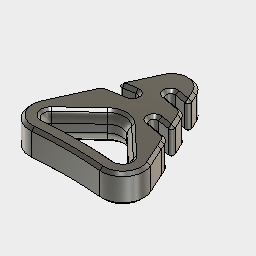
GuylineQuickAdjuster (Autodesk Fusion 360 design; units mm, degrees)
Autodesk Fusion 360 part; units mm, degrees
sketch "Sketch1" plane through (0, 0, 0) normal (0, 0, 1) x (1, 0, 0)
  line L0 (6.8861, 1.5182) -> (1.7133, 6.3871)
  line L1 (8.5, 0) -> (18.6301, 0) construction
  line L2 (-6.8869, 1.5182) -> (-1.7136, 6.3872)
  arc A0 (6.3068, 0.2249) -> (-6.3077, 0.2249) centre (-0.0001, -72) ccw
  arc A1 (-6.8869, 1.5182) -> (-6.3077, 0.2249) centre (-6.3729, 0.972) ccw
  arc A2 (6.3068, 0.2249) -> (6.8861, 1.5182) centre (6.372, 0.9721) ccw
  arc A3 (1.7133, 6.3871) -> (-1.7136, 6.3872) centre (-0.0002, 4.5667) ccw
  arc A4 (-9.7878, 2.5199) -> (-6.0467, -2.7631) centre (-6.3729, 0.972) ccw
  arc A5 (6.0459, -2.763) -> (-6.0467, -2.7631) centre (-0.0001, -72) ccw
  arc A6 (6.0459, -2.763) -> (9.7871, 2.5196) centre (6.372, 0.9721) ccw
  line L3 (-0.0001, 7.0667) -> (-0.0001, 7.5)
  line L4 (-0.0001, 7.0667) -> (-0.0027, 10.0001) construction
  line L5 (-0.0027, 10.0001) -> (-0.0001, 12.0001) construction
  line L6 (-0.0001, 12.0001) -> (0.0118, 15.0001) construction
  line L7 (0.0118, 15.0001) -> (6.9911, 13.7685) construction
  line L8 (-0.0027, 10.0001) -> (11.5438, 7.9642) construction
  line L9 (-0.0027, 10.0001) -> (11.5483, 10.0001) construction
  line L10 (-0.0001, 12.0001) -> (-12.6146, 9.7758) construction
  line L11 (-0.0001, 12.0001) -> (12.8092, 12.0001) construction
  line L12 (-4.6584, 11.9394) -> (-2.6377, 12.2955)
  line L13 (-2.3804, 10.8188) -> (-5.3051, 10.3031)
  line L14 (-6.7795, 9.159) -> (-9.7878, 2.5199)
  line L15 (8.2551, 5.8972) -> (9.7871, 2.5196)
  line L16 (-0.1302, 14.2615) -> (0, 14.2386)
  line L17 (0.9018, 14.0794) -> (3.819, 13.5647)
  arc A7 (-2.3804, 10.8188) -> (-2.6377, 12.2955) centre (-2.5076, 11.5574) ccw
  arc A8 (-5.2006, 12.6383) -> (-4.6584, 11.9394) centre (-4.7452, 12.4318) ccw
  arc A9 (-5.3051, 10.3031) -> (-6.7795, 9.159) centre (-4.9578, 8.3335) ccw
  arc A10 (5.2925, 12.4219) -> (3.819, 13.5647) centre (3.4715, 11.5951) ccw
  line L18 (5.6391, 9.7659) -> (3.6186, 10.1215)
  line L19 (5.2925, 12.4219) -> (6.1811, 10.465)
  line L20 (7.7598, 6.988) -> (8.2551, 5.8972)
  line L21 (3.3647, 8.6452) -> (6.2855, 8.1309)
  arc A11 (3.6186, 10.1215) -> (3.3647, 8.6452) centre (3.4887, 9.3839) ccw
  arc A12 (5.6391, 9.7659) -> (6.1811, 10.465) centre (5.7258, 10.2583) ccw
  arc A13 (7.7598, 6.988) -> (6.2855, 8.1309) centre (5.9387, 6.1612) ccw
  line L22 (3.1695, 15.2045) -> (1.1628, 15.5586)
  arc A14 (1.1628, 15.5586) -> (0.9558, 14.0699) centre (1.0321, 14.818) ccw
  line L23 (3.7117, 15.9036) -> (3.041, 17.3808)
  line L24 (-5.2006, 12.6383) -> (-3.0395, 17.3841)
  arc A15 (3.041, 17.3808) -> (-3.0395, 17.3841) centre (0, 16) ccw
  arc A16 (3.1695, 15.2045) -> (3.7117, 15.9036) centre (3.2564, 15.6968) ccw
  line L25 (0.1421, 15.7387) -> (7.1214, 14.5071) construction
  point P0 (-5.5922, 11.7748)
  point P1 (7.0718, 8.5146)
  point P2 (6.5732, 9.6014)
  dimension "d4" = 0.75
  dimension "d5" = 0.75
  dimension "d6" = 2.5
  dimension "d13" = 2
  dimension "d14" = 3
  dimension "d16" = 10
  dimension "d17" = 170
  dimension "d24" = 3
  dimension "d30" = 0.5
  dimension "d31" = 2
  dimension "d33" = 2
  dimension "d41" = 3
  dimension "d42" = 0.5
  dimension "d43" = 2
  dimension "d44" = 0.75
  dimension "d45" = 0.5
  measures "d4" radius of A1
  measures "d5" radius of A2
  measures "d6" radius of A3
  measures "d13" distance of L4.end L5.end
  measures "d14" distance of L5.end L6.end
  measures "d16" angle of L8 L9
  measures "d17" angle of L10 L11
  measures "d24" distance of P0 L12.end
  measures "d30" radius of A8
  measures "d31" radius of A9
  measures "d33" radius of A10
  measures "d41" distance of P2 L18.end
  measures "d42" radius of A12
  measures "d43" radius of A13
  measures "d45" radius of A16
extrude "Extrude1" add sketch "Sketch1" along normal blind 5
chamfer "Chamfer1" distance 0.5 angle 45 50 edges at (-3.8428, 10.561, 5) (-6.1839, 9.9136, 5) (-8.2836, 5.8394, 5) (-9.4327, -1.1947, 5) (-0.0004, -2.4995, 5) (9.4317, -1.1948, 5) (9.0211, 4.2084, 5) (8.0074, 6.4426, 5) (7.1641, 7.7419, 5) (4.8251, 8.388, 5) (-3.8428, 10.561, 0) (-6.1839, 9.9136, 0) (-8.2836, 5.8394, 0) (-9.4327, -1.1947, 0) (-0.0004, -2.4995, 0) (9.4317, -1.1948, 0) (9.0211, 4.2084, 0) (8.0074, 6.4426, 0) (7.1641, 7.7419, 0) (4.8251, 8.388, 0) (2.7505, 9.5108, 5) (4.6289, 9.9437, 5) (6.121, 9.952, 5) (5.7368, 11.4435, 5) (4.6971, 13.1755, 5) (2.3874, 13.8173, 5) (0.2872, 14.9216, 5) (2.1662, 15.3815, 5) (3.6515, 15.3904, 5) (3.3763, 16.6422, 5) (0.0018, 19.3398, 5) (-4.12, 15.0112, 5) (-5.1403, 12.1254, 5) (-3.6481, 12.1175, 5) (-1.7692, 11.6861, 5) (2.3874, 13.8173, 0) (4.6971, 13.1755, 0) (5.7368, 11.4435, 0) (6.121, 9.952, 0) (4.6289, 9.9437, 0) (2.7505, 9.5108, 0) (-1.7692, 11.6861, 0) (-3.6481, 12.1175, 0) (-5.1403, 12.1254, 0) (-4.12, 15.0112, 0) (0.0018, 19.3398, 0) (3.3763, 16.6422, 0) (3.6515, 15.3904, 0) (2.1662, 15.3815, 0) (0.2872, 14.9216, 0)
chamfer "Chamfer2" distance 1 angle 45 6 edges at (7.0565, 0.6655, 5) (-0.0004, 0.4998, 5) (-7.0574, 0.6654, 5) (-4.3003, 3.9527, 5) (-0.0001, 7.0667, 5) (4.2997, 3.9527, 5)
chamfer "Chamfer3" distance 1 angle 45 6 edges at (7.0565, 0.6655, 0) (-0.0004, 0.4998, 0) (-7.0574, 0.6654, 0) (-4.3003, 3.9527, 0) (-0.0001, 7.0667, 0) (4.2997, 3.9527, 0)
fillet "Fillet1" radius 2 12 edges at (7.0565, 0.6655, 4) (-0.0004, 0.4998, 4) (-7.0574, 0.6654, 4) (-4.3003, 3.9527, 4) (-0.0001, 7.0667, 4) (4.2997, 3.9527, 4) (-7.0574, 0.6654, 1) (-0.0004, 0.4998, 1) (7.0565, 0.6655, 1) (4.2997, 3.9527, 1) (-0.0001, 7.0667, 1) (-4.3003, 3.9527, 1)
